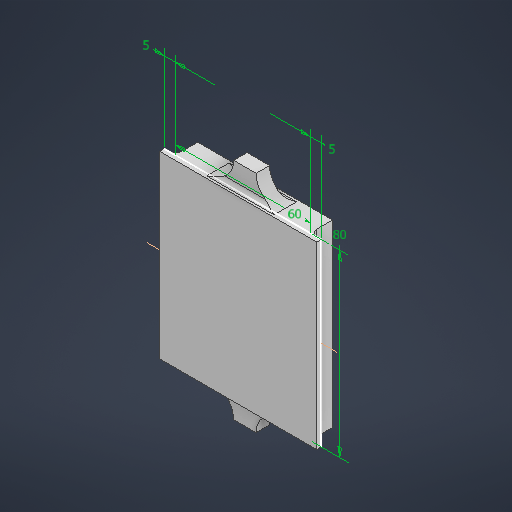
# Autodesk Inventor part: Repetidor
Saved by Autodesk Inventor 2026.2 (Build 302298010, 298A)
## iProperties
Created: 2026-04-26
Part Number: Repetidor
Material: Genérico
Document SubType Name: Modeling
Designer: Lucas David
Density: 1 g/cm^3
Appearance: Padrão
Author: Lucas David
Autodesk Inventor part; units mm, degrees
ref_plane "YZ Plane" through (0, 0, 0) normal (1, 0, 0) x (0, 1, 0)
ref_plane "XZ Plane" through (0, 0, 0) normal (0, 1, 0) x (-1, 0, 0)
ref_plane "XY Plane" through (0, 0, 0) normal (0, 0, 1) x (1, 0, 0)
sketch "Esboço1" plane through (0, 0, 0) normal (0, 0, 1) x (1, 0, 0)
  line L0 (-30, -40) -> (30, -40)
  line L1 (30, -40) -> (30, 40)
  line L2 (30, 40) -> (-30, 40)
  line L3 (-30, 40) -> (-30, -40)
  line L4 (-30, -40) -> (30, 40) construction
  line L5 (30, -40) -> (-30, 40) construction
  line L6 (35, 40) -> (35, -40)
  line L7 (-35, -40) -> (-35, 40)
  line L8 (30, -40) -> (35, -40)
  line L9 (-35, -40) -> (-30, -40)
  line L10 (-35, 40) -> (-30, 40)
  line L11 (30, 40) -> (35, 40)
  point P0 (0, 0)
  dimension "d0" = 60
  dimension "d1" = 80
  dimension "d2" = 5
  dimension "d3" = 5
  constraints: 24 end point, 4 point on line, 3 horizontal, 3 parallel, 2 midpoint, 2 perpendicular, 1 collinear
  measures "d0" distance between parallel lines of L1 L3
  measures "d1" distance between parallel lines of L0 L2
  measures "d2" distance between parallel lines of L6 L1
  measures "d3" distance between parallel lines of L3 L7
extrude "Extrusão1" add sketch "Esboço1" along normal blind 2
extrude "Extrusão2" add sketch "Esboço1" against normal blind 10 contours L3 L2 L1 L0
fillet "Arredondamento1" radius 3 2 edges at (30, 0, 0) (-30, 0, 0)
sketch "Esboço2" plane through (-35, -40, 2) normal (0, -1, 0) x (1, 0, 0)
  line L0 (65, -12) -> (5, -12) projected
  line L1 (65, -12) -> (65, 0)
  line L2 (0, 0) -> (70, 0) projected
  line L3 (65, -6) -> (5, -6) construction
  line L4 (5, -5) -> (5, -12) projected
  line L5 (40, -3) -> (30, -3)
  line L6 (30, -3) -> (30, -9)
  line L7 (30, -9) -> (40, -9)
  line L8 (40, -9) -> (40, -3)
  line L9 (40, -3) -> (30, -9) construction
  line L10 (30, -3) -> (40, -9) construction
  point P0 (35, -2)
  point P1 (35, -6)
  dimension "d9" = 10
  dimension "d10" = 6
  constraints: 16 end point, 4 midpoint, 2 horizontal, 2 parallel, 2 point on line, 1 perpendicular, 1 vertical
  measures "d9" distance between parallel lines of L6 L8
  measures "d10" distance between parallel lines of L5 L7
extrude "Extrusão3" add sketch "Esboço2" along normal blind 10
fillet "Arredondamento2" radius 10 2 edges at (5, -40, -4) (-5, -40, -4)
fillet "Arredondamento3" radius 2 2 edges at (0, -40, -7) (0, -40, -1)
mirror "Espelhar1" about plane through (0, 0, 0) normal (0, 1, 0) of "Arredondamento2", "Extrusão3", "Arredondamento3"
